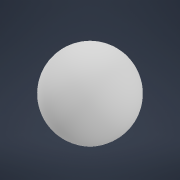
# Autodesk Inventor part: 16
Saved by Autodesk Inventor 2021.2 (Build 252289000, 289)
## iProperties
Created: 2023-09-07
Part Number: 16
Material: Типовые
Document SubType Name: Modeling
Designer: User
Density: 1 g/cm^3
Appearance: По умолчанию
Author: User
Autodesk Inventor part; units mm, degrees
ref_plane "YZ Plane" through (0, 0, 0) normal (1, 0, 0) x (0, 1, 0)
ref_plane "XZ Plane" through (0, 0, 0) normal (0, 1, 0) x (-1, 0, 0)
ref_plane "XY Plane" through (0, 0, 0) normal (0, 0, 1) x (1, 0, 0)
sketch "Эскиз1" plane through (0, 0, 0) normal (0, 0, 1) x (1, 0, 0)
  line L0 (-4.9749, -7.5) -> (-2, -7.5)
  arc A0 (-9, 0) -> (-4.9749, -7.5) centre (0, 0) ccw
  arc A1 (0, 9) -> (-9, 0) centre (0, 0) ccw
  line L1 (-2, -7.5) -> (-2, -3.8)
  line L2 (-2, -3.8) -> (0, -3.8)
  line L3 (0, 9) -> (0, -3.8)
  dimension "d4" = 3.7
  dimension "d5" = 16.5
  dimension "d6" = 9
  constraints: 8 end point, 4 point on circle, 2 centre point, 1 coincident, 1 horizontal
  measures "d4" distance of L0.end L1.end
  measures "d6" radius of A1
revolve "Вращение1" add sketch "Эскиз1" angle 360 about axis through (0, 9, 0) along (0, -1, 0)
